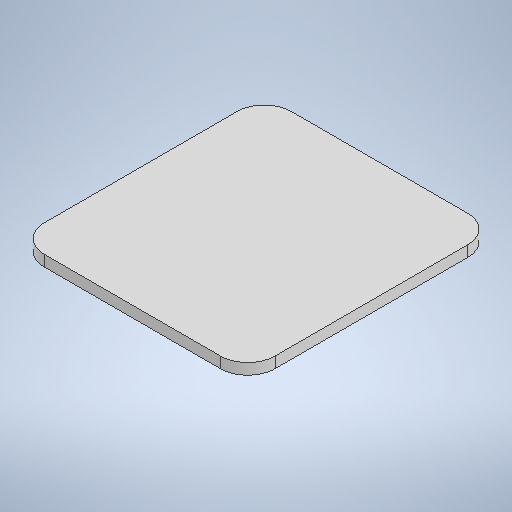
# Autodesk Inventor part: PCB_Mount
Saved by Autodesk Inventor 2025.2 (Build 292293000, 293)
## iProperties
Created: 2024-11-12
Part Number: PCB_Mount
Material: Generic
Document SubType Name: Modeling
Designer: matss
Density: 1 g/cm^3
Appearance: Default
Author: matss
Autodesk Inventor part; units mm, degrees
ref_plane "YZ Plane" through (0, 0, 0) normal (1, 0, 0) x (0, 1, 0)
ref_plane "XZ Plane" through (0, 0, 0) normal (0, 1, 0) x (-1, 0, 0)
ref_plane "XY Plane" through (0, 0, 0) normal (0, 0, 1) x (1, 0, 0)
sketch "Sketch1" plane through (0, 0, 0) normal (0, 1, 0) x (-1, 0, 0)
  line L0 (0, 14.23) -> (0, -14.23) construction
  circle A0 centre (0, 14.23) radius 1
  circle A1 centre (0, -14.23) radius 1
  line L1 (8, 22.5) -> (-34, 22.5)
  line L2 (-34, 22.5) -> (-34, -22.5)
  line L3 (-34, -22.5) -> (8, -22.5)
  line L4 (8, -22.5) -> (8, 22.5)
  point P0 (0, 0)
  point P1 (0, 0)
  point P2 (8, 0)
  dimension "d0" = 28.46
  dimension "d1" = 2
  dimension "d2" = 2
  dimension "d3" = 45
  dimension "d4" = 42
  dimension "d5" = 8
  constraints: 10 end point, 3 coincident, 2 centre point, 2 midpoint, 2 parallel, 1 horizontal, 1 horizontal alignment, 1 perpendicular
  measures "d0" distance of L0.start L0.end
  measures "d1" diameter of A0
  measures "d2" diameter of A1
  measures "d3" distance of L3.end L1.start
  measures "d4" distance between parallel lines of L2 L4
  measures "d5" distance between parallel lines of L0 L4
extrude "Extrusion1" add sketch "Sketch1" along normal blind 2 contours A0 | A1 | L4 L3 L2 L1
extrude "Extrusion2" add sketch "Sketch1" against normal blind 5 contours A0 | A1
sketch "Sketch2" plane through (0, 0, 0) normal (0, -1, 0) x (1, 0, 0)
  line L0 (20, -7.5) -> (25, -7.5)
  line L1 (25, -7.5) -> (25, -2.5)
  line L2 (25, -2.5) -> (20, -2.5)
  line L3 (20, -2.5) -> (20, -7.5)
  line L4 (34, 22.5) -> (34, -22.5) projected
  line L5 (34, -22.5) -> (-8, -22.5) projected
  point P0 (0, 0)
  dimension "d10" = 5
  dimension "d11" = 5
  dimension "d12" = 9
  dimension "d13" = 15
  constraints: 8 end point, 2 parallel, 1 horizontal, 1 perpendicular
  measures "d10" distance of L2.end L0.start
  measures "d11" distance of L0.start L0.end
  measures "d12" distance between parallel lines of L4 L1
  measures "d13" distance between parallel lines of L5 L0
extrude "Extrusion3" add sketch "Sketch2" along normal blind 2.5
sketch "Sketch3" plane through (0, 0, 0) normal (0, -1, 0) x (1, 0, 0)
  line L0 (-1, -5) -> (1, -5)
  line L1 (1, -5) -> (1, 5)
  line L2 (1, 5) -> (-1, 5)
  line L3 (-1, 5) -> (-1, -5)
  circle A0 centre (0, 14.23) radius 1 projected
  circle A1 centre (0, -14.23) radius 1 projected
  circle A2 centre (0, 14.23) radius 1 projected
  circle A3 centre (0, -14.23) radius 1 projected
  point P0 (0, 0)
  point P1 (0, -5)
  point P2 (-1, 0)
  dimension "d16" = 2
  dimension "d17" = 10
  constraints: 8 end point, 2 midpoint, 2 parallel, 1 horizontal, 1 horizontal alignment, 1 perpendicular, 1 vertical alignment
  measures "d16" distance of L1.end L2.end
  measures "d17" distance of L2.end L0.start
extrude "Extrusion4" add sketch "Sketch3" along normal blind 2.5 contours L3 L2 L1 L0
fillet "Fillet1" radius 0.5 8 edges at (-1, -1.25, -5) (1, -1.25, -5) (1, -1.25, 5) (-1, -1.25, 5) (20, -1.25, -7.5) (20, -1.25, -2.5) (25, -1.25, -7.5) (25, -1.25, -2.5)
chamfer "Chamfer2" distance 0.5 angle 45 2 edges at (1, 0, -14.23) (1, 0, 14.23)
fillet "Fillet2" radius 5 4 edges at (34, 1, -22.5) (34, 1, 22.5) (-8, 1, 22.5) (-8, 1, -22.5)
body "Solid1"
